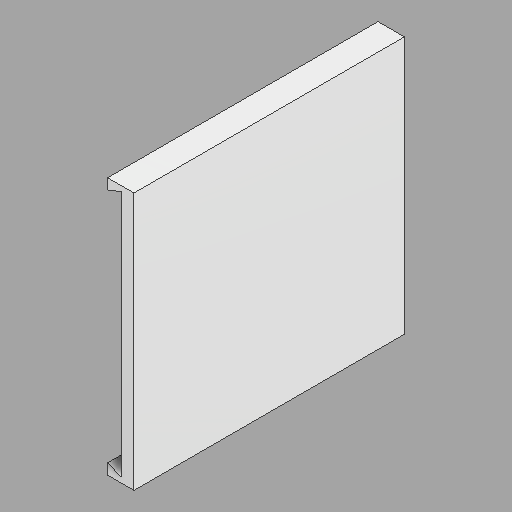
# Autodesk Inventor part: door3
Saved by Autodesk Inventor 2025.2 (Build 292293000, 293)
## iProperties
Created: 2025-02-23
Part Number: door3
Material: ABS Plastic
Document SubType Name: Modeling
Designer: Alex
Density: 1.06 g/cm^3
Appearance: Smooth - White
Author: Alex
Autodesk Inventor part; units mm, degrees
ref_plane "YZ Plane" through (0, 0, 0) normal (1, 0, 0) x (0, 1, 0)
ref_plane "XZ Plane" through (0, 0, 0) normal (0, 1, 0) x (-1, 0, 0)
ref_plane "XY Plane" through (0, 0, 0) normal (0, 0, 1) x (1, 0, 0)
sketch "Sketch1" plane through (0, 0, 0) normal (0, 0, 1) x (1, 0, 0)
  line L0 (49.8, 1.2046) -> (44.8, -0.7954) construction
  line L1 (44.8, -0.7954) -> (44.8, 3.5) construction
  line L2 (44.8, 3.5) -> (-50, 3.5) construction
  line L3 (-50, 3.5) -> (-50, -0.5) construction
  line L4 (-50, -0.5) -> (-45, 1.5) construction
  line L5 (-45, 1.5) -> (-45, -3.5) construction
  line L6 (-45, -3.5) -> (49.8, -3.5) construction
  line L7 (44.8, -92.2046) -> (49.8, -94.2046) construction
  line L8 (49.8, -89.5) -> (-45, -89.5) construction
  line L9 (-45, -89.5) -> (-45, -94.5) construction
  line L10 (-45, -94.5) -> (-50, -92.5) construction
  line L11 (-50, -92.5) -> (-50, -96.5) construction
  line L12 (-50, -96.5) -> (44.8, -96.5) construction
  line L13 (44.8, -96.5) -> (44.8, -92.2046) construction
  line L14 (44.9, 3.5) -> (44.9, -0.6477)
  line L15 (44.9, -0.6477) -> (50.15, 1.4523)
  line L16 (44.9, 3.5) -> (55.15, 3.5)
  line L17 (55.15, 3.5) -> (55.15, -96.5)
  line L18 (55.15, -96.5) -> (44.9, -96.5)
  line L19 (44.9, -96.5) -> (44.9, -92.3523)
  line L20 (44.9, -92.3523) -> (50.15, -94.4523)
  line L21 (50.15, -94.4523) -> (50.15, 1.4523)
  line L22 (49.8, -94.2046) -> (49.8, -89.5) projected
  line L23 (49.8, -3.5) -> (49.8, 1.2046) projected
  point P0 (0, 0)
  dimension "d0" = 0.1
  dimension "d1" = 0.1
  dimension "d3" = 5
  constraints: 16 end point, 5 parallel, 2 collinear, 2 equal length, 2 perpendicular, 1 horizontal, 1 vertical
  measures "d0" distance between parallel lines of L0 L15
  measures "d1" distance between parallel lines of L1 L14
  measures "d3" distance between parallel lines of L17 L21
extrude "Extrusion1" add sketch "Sketch1" against normal blind 100
sketch "Sketch2" plane through (0, 0, -100) normal (0, 0, -1) x (-1, 0, 0)
  line L0 (-44.9, -0.6477) -> (-44.9, 3.5) projected
  line L1 (-55.15, 3.5) -> (-55.15, -96.5) projected
  line L2 (-44.9, 3.5) -> (-55.15, 3.5)
  line L3 (-55.15, 3.5) -> (-55.15, -96.5)
  line L4 (-55.15, -96.5) -> (-44.9, -96.5)
  line L5 (-44.9, -96.5) -> (-44.9, 3.5)
  point P0 (0, 0)
  constraints: 8 end point, 2 parallel, 1 horizontal, 1 perpendicular
extrude "Extrusion2" add sketch "Sketch2" along normal blind 5
sketch "Sketch3" plane through (50.15, -94.4523, 0) normal (0.3713907, 0.9284767, 0) x (0.9284767, -0.3713907, 0)
  circle A0 centre (-2.8272, 90) radius 1
  line L0 (-5.6544, 100) -> (0, 100) construction
  line L1 (-2.8272, 100) -> (-2.8272, 90) construction
  point P0 (-81.6418, 0)
  dimension "d8" = 2
  dimension "d9" = 10
  constraints: 2 end point, 1 centre point, 1 midpoint, 1 perpendicular
  measures "d8" diameter of A0
  measures "d9" distance of L1.start L1.end
extrude "Extrusion3" cut sketch "Sketch3" against normal blind 0.5
fillet "Fillet1" radius 1 2 edges at (46.4101, -93.497, -90) (46.5965, -93.0309, -90)
body "Solid1"
